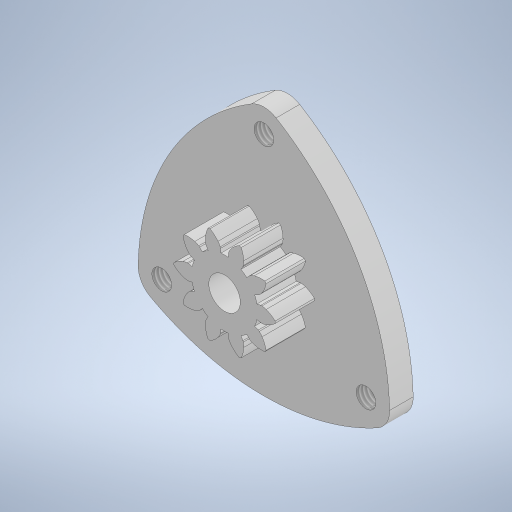
# Autodesk Inventor part: 多段ギアm2z10t8
Saved by Autodesk Inventor 2023 (Build 270158000, 158)
## iProperties
Created: 2022-01-10
Part Number: 多段ギアm2z10t8
Material: Generic
Document SubType Name: Modeling
Designer: acps
Density: 1 g/cm^3
Appearance: Default
Author: acps
Autodesk Inventor part; units mm, degrees
ref_plane "YZ Plane" through (0, 0, 0) normal (1, 0, 0) x (0, 1, 0)
ref_plane "XZ Plane" through (0, 0, 0) normal (0, 1, 0) x (-1, 0, 0)
ref_plane "XY Plane" through (0, 0, 0) normal (0, 0, 1) x (1, 0, 0)
sketch "Sketch1" plane through (0, 0, 0) normal (0, 0, 1) x (1, 0, 0)
  circle A0 centre (0, 0) radius 2
  arc A1 (0.5556, 4.8181) -> (0.5131, 4.6704) centre (1.1772, 4.5593) ccw
  arc A2 (0.8331, 5.2927) -> (0.5556, 4.8181) centre (2.3167, 4.1066) ccw
  arc A3 (1.8568, 6.1598) -> (0.8331, 5.2927) centre (3.5506, 3.1222) ccw
  arc A4 (-2.3825, 4.2245) -> (-2.3301, 4.08) centre (-1.7275, 4.3805) ccw
  arc A5 (-2.437, 4.7715) -> (-2.3825, 4.2245) centre (-0.5396, 4.6841) ccw
  arc A6 (-2.1184, 6.0748) -> (-2.437, 4.7715) centre (1.0373, 4.6129) ccw
  arc A7 (-4.4106, 2.0173) -> (-4.2832, 1.9312) centre (-3.9723, 2.5285) ccw
  arc A8 (-4.7762, 2.4278) -> (-4.4106, 2.0173) centre (-3.1898, 3.4723) ccw
  arc A9 (-5.2845, 3.6694) -> (-4.7762, 2.4278) centre (-1.8722, 4.3416) ccw
  arc A10 (-4.754, -0.9605) -> (-4.6003, -0.9553) centre (-4.6999, -0.2893) ccw
  arc A11 (-5.2911, -0.8432) -> (-4.754, -0.9605) centre (-4.6215, 0.9343) ccw
  arc A12 (-6.4321, -0.1375) -> (-5.2911, -0.8432) centre (-4.0666, 2.412) ccw
  arc A13 (-3.2815, -3.5714) -> (-3.1603, -3.4768) centre (-3.6323, -2.9966) ccw
  arc A14 (-3.7849, -3.7922) -> (-3.2815, -3.5714) centre (-4.2881, -1.9606) ccw
  arc A15 (-5.1228, -3.892) -> (-3.7849, -3.7922) centre (-4.7077, -0.439) ccw
  arc A16 (-0.5556, -4.8181) -> (-0.5131, -4.6704) centre (-1.1772, -4.5593) ccw
  arc A17 (-0.8331, -5.2927) -> (-0.5556, -4.8181) centre (-2.3167, -4.1066) ccw
  arc A18 (-1.8568, -6.1598) -> (-0.8331, -5.2927) centre (-3.5506, -3.1222) ccw
  arc A19 (2.3825, -4.2245) -> (2.3301, -4.08) centre (1.7275, -4.3805) ccw
  arc A20 (2.437, -4.7715) -> (2.3825, -4.2245) centre (0.5396, -4.6841) ccw
  arc A21 (2.1184, -6.0748) -> (2.437, -4.7715) centre (-1.0373, -4.6129) ccw
  arc A22 (4.4106, -2.0173) -> (4.2832, -1.9312) centre (3.9723, -2.5285) ccw
  arc A23 (4.7762, -2.4278) -> (4.4106, -2.0173) centre (3.1898, -3.4723) ccw
  arc A24 (5.2845, -3.6694) -> (4.7762, -2.4278) centre (1.8722, -4.3416) ccw
  arc A25 (4.754, 0.9605) -> (4.6003, 0.9553) centre (4.6999, 0.2893) ccw
  arc A26 (5.2911, 0.8432) -> (4.754, 0.9605) centre (4.6215, -0.9343) ccw
  arc A27 (6.4321, 0.1375) -> (5.2911, 0.8432) centre (4.0666, -2.412) ccw
  arc A28 (3.2815, 3.5714) -> (3.1603, 3.4768) centre (3.6323, 2.9966) ccw
  arc A29 (3.7849, 3.7922) -> (3.2815, 3.5714) centre (4.2881, 1.9606) ccw
  arc A30 (5.1228, 3.892) -> (3.7849, 3.7922) centre (4.7077, 0.439) ccw
  arc A31 (-0.5131, 4.6704) -> (-0.5556, 4.8181) centre (-1.1772, 4.5593) ccw
  arc A32 (-0.5556, 4.8181) -> (-0.8331, 5.2927) centre (-2.3167, 4.1066) ccw
  arc A33 (-0.8331, 5.2927) -> (-1.8568, 6.1598) centre (-3.5506, 3.1222) ccw
  arc A34 (-3.1603, 3.4768) -> (-3.2815, 3.5714) centre (-3.6323, 2.9966) ccw
  arc A35 (-3.2815, 3.5714) -> (-3.7849, 3.7922) centre (-4.2881, 1.9606) ccw
  arc A36 (-3.7849, 3.7922) -> (-5.1228, 3.892) centre (-4.7077, 0.439) ccw
  arc A37 (-4.6003, 0.9553) -> (-4.754, 0.9605) centre (-4.6999, 0.2893) ccw
  arc A38 (-4.754, 0.9605) -> (-5.2911, 0.8432) centre (-4.6215, -0.9343) ccw
  arc A39 (-5.2911, 0.8432) -> (-6.4321, 0.1375) centre (-4.0666, -2.412) ccw
  arc A40 (-4.2832, -1.9312) -> (-4.4106, -2.0173) centre (-3.9723, -2.5285) ccw
  arc A41 (-4.4106, -2.0173) -> (-4.7762, -2.4278) centre (-3.1898, -3.4723) ccw
  arc A42 (-4.7762, -2.4278) -> (-5.2845, -3.6694) centre (-1.8722, -4.3416) ccw
  arc A43 (-2.3301, -4.08) -> (-2.3825, -4.2245) centre (-1.7275, -4.3805) ccw
  arc A44 (-2.3825, -4.2245) -> (-2.437, -4.7715) centre (-0.5396, -4.6841) ccw
  arc A45 (-2.437, -4.7715) -> (-2.1184, -6.0748) centre (1.0373, -4.6129) ccw
  arc A46 (0.5131, -4.6704) -> (0.5556, -4.8181) centre (1.1772, -4.5593) ccw
  arc A47 (0.5556, -4.8181) -> (0.8331, -5.2927) centre (2.3167, -4.1066) ccw
  arc A48 (0.8331, -5.2927) -> (1.8568, -6.1598) centre (3.5506, -3.1222) ccw
  arc A49 (3.1603, -3.4768) -> (3.2815, -3.5714) centre (3.6323, -2.9966) ccw
  arc A50 (3.2815, -3.5714) -> (3.7849, -3.7922) centre (4.2881, -1.9606) ccw
  arc A51 (3.7849, -3.7922) -> (5.1228, -3.892) centre (4.7077, -0.439) ccw
  arc A52 (4.6003, -0.9553) -> (4.754, -0.9605) centre (4.6999, -0.2893) ccw
  arc A53 (4.754, -0.9605) -> (5.2911, -0.8432) centre (4.6215, 0.9343) ccw
  arc A54 (5.2911, -0.8432) -> (6.4321, -0.1375) centre (4.0666, 2.412) ccw
  arc A55 (4.2832, 1.9312) -> (4.4106, 2.0173) centre (3.9723, 2.5285) ccw
  arc A56 (4.4106, 2.0173) -> (4.7762, 2.4278) centre (3.1898, 3.4723) ccw
  arc A57 (4.7762, 2.4278) -> (5.2845, 3.6694) centre (1.8722, 4.3416) ccw
  arc A58 (2.3301, 4.08) -> (2.3825, 4.2245) centre (1.7275, 4.3805) ccw
  arc A59 (2.3825, 4.2245) -> (2.437, 4.7715) centre (0.5396, 4.6841) ccw
  arc A60 (2.437, 4.7715) -> (2.1184, 6.0748) centre (-1.0373, 4.6129) ccw
  arc A61 (0.4586, 4.1749) -> (-0.4586, 4.1749) centre (0, 0) ccw
  arc A62 (-2.0829, 3.6471) -> (-2.825, 3.108) centre (0, 0) ccw
  arc A63 (-3.8288, 1.7263) -> (-4.1123, 0.8539) centre (0, 0) ccw
  arc A64 (-4.1123, -0.8539) -> (-3.8288, -1.7263) centre (0, 0) ccw
  arc A65 (-2.825, -3.108) -> (-2.0829, -3.6471) centre (0, 0) ccw
  arc A66 (-0.4586, -4.1749) -> (0.4586, -4.1749) centre (0, 0) ccw
  arc A67 (2.0829, -3.6471) -> (2.825, -3.108) centre (0, 0) ccw
  arc A68 (3.8288, -1.7263) -> (4.1123, -0.8539) centre (0, 0) ccw
  arc A69 (4.1123, 0.8539) -> (3.8288, 1.7263) centre (0, 0) ccw
  arc A70 (2.825, 3.108) -> (2.0829, 3.6471) centre (0, 0) ccw
  arc A71 (-1.8568, 6.1598) -> (-2.1184, 6.0748) centre (0, 0) ccw
  arc A72 (-5.1228, 3.892) -> (-5.2845, 3.6694) centre (0, 0) ccw
  arc A73 (-6.4321, 0.1375) -> (-6.4321, -0.1375) centre (0, 0) ccw
  arc A74 (-5.2845, -3.6694) -> (-5.1228, -3.892) centre (0, 0) ccw
  arc A75 (-2.1184, -6.0748) -> (-1.8568, -6.1598) centre (0, 0) ccw
  arc A76 (1.8568, -6.1598) -> (2.1184, -6.0748) centre (0, 0) ccw
  arc A77 (5.1228, -3.892) -> (5.2845, -3.6694) centre (0, 0) ccw
  arc A78 (6.4321, -0.1375) -> (6.4321, 0.1375) centre (0, 0) ccw
  arc A79 (5.2845, 3.6694) -> (5.1228, 3.892) centre (0, 0) ccw
  arc A80 (2.1184, 6.0748) -> (1.8568, 6.1598) centre (0, 0) ccw
  line L0 (0.4586, 4.1749) -> (0.5131, 4.6704)
  line L1 (-2.0829, 3.6471) -> (-2.3301, 4.08)
  line L2 (-3.8288, 1.7263) -> (-4.2832, 1.9312)
  line L3 (-4.1123, -0.8539) -> (-4.6003, -0.9553)
  line L4 (-2.825, -3.108) -> (-3.1603, -3.4768)
  line L5 (-0.4586, -4.1749) -> (-0.5131, -4.6704)
  line L6 (2.0829, -3.6471) -> (2.3301, -4.08)
  line L7 (3.8288, -1.7263) -> (4.2832, -1.9312)
  line L8 (4.1123, 0.8539) -> (4.6003, 0.9553)
  line L9 (2.825, 3.108) -> (3.1603, 3.4768)
  line L10 (-0.4586, 4.1749) -> (-0.5131, 4.6704)
  line L11 (-2.825, 3.108) -> (-3.1603, 3.4768)
  line L12 (-4.1123, 0.8539) -> (-4.6003, 0.9553)
  line L13 (-3.8288, -1.7263) -> (-4.2832, -1.9312)
  line L14 (-2.0829, -3.6471) -> (-2.3301, -4.08)
  line L15 (0.4586, -4.1749) -> (0.5131, -4.6704)
  line L16 (2.825, -3.108) -> (3.1603, -3.4768)
  line L17 (4.1123, -0.8539) -> (4.6003, -0.9553)
  line L18 (3.8288, 1.7263) -> (4.2832, 1.9312)
  line L19 (2.0829, 3.6471) -> (2.3301, 4.08)
  dimension "d34" = 4
  constraints: 160 point on circle, 81 centre point, 40 end point, 1 coincident
  measures "d34" diameter of A0
extrude "Extrusion1" add sketch "Sketch1" along normal blind 5
sketch "Sketch3" plane through (0, 0, 0) normal (0, 0, -1) x (-1, 0, 0)
  circle A0 centre (-12.9904, -7.5) radius 1.25
  circle A1 centre (12.9904, -7.5) radius 1.25
  circle A2 centre (0, 15) radius 1.25
  circle A3 centre (0, 0) radius 20.05 construction
  circle A4 centre (0, 0) radius 18.25 construction
  circle A5 centre (-12.9904, -7.5) radius 3.25 construction
  circle A6 centre (-12.9904, -7.5) radius 3
  circle A7 centre (12.9904, -7.5) radius 3
  circle A8 centre (0, 15) radius 3
  arc A9 (-1.5559, 17.565) -> (-15.9897, -7.435) centre (14.0033, -8.0848) ccw
  arc A10 (-14.4338, -10.13) -> (14.4338, -10.13) centre (0, 16.1696) ccw
  arc A11 (15.9897, -7.435) -> (1.5559, 17.565) centre (-14.0033, -8.0848) ccw
  circle A12 centre (0, 0) radius 2
  point P0 (15.9897, -7.435)
  point P1 (1.5559, 17.565)
  point P2 (-14.4338, -10.13)
  point P3 (14.4338, -10.13)
  dimension "d14" = 6
  dimension "d18" = 6
  dimension "d3" = 2.5
  dimension "d6" = 360
  dimension "d9" = 40.1
  dimension "d10" = 36.5
  dimension "d11" = 6.5
  dimension "d17" = 6
  dimension "d19" = 30
  dimension "d22" = 360
  dimension "d33" = 4
  constraints: 11 centre point, 7 coincident, 6 point on circle, 1 horizontal alignment, 1 tangent, 28 other
  measures "d3" diameter of A0
  measures "d9" diameter of A3
  measures "d10" diameter of A4
  measures "d11" diameter of A5
  measures "d17" diameter of A7
  measures "d19" radius of A9
  measures "d33" diameter of A12
extrude "Extrusion2" add sketch "Sketch3" along normal blind 3
thread "Thread1" size "M3x0.5" class "6H" standard "ANSI Metric M Profile" full length
thread "Thread2" size "M3x0.5" class "6H" standard "ANSI Metric M Profile" full length
thread "Thread3" size "M3x0.5" class "6H" standard "ANSI Metric M Profile" full length
body "Solid1"
